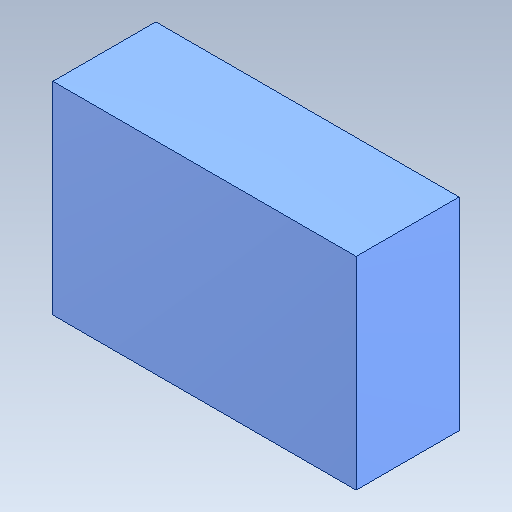
# Autodesk Inventor part: 100
Saved by Autodesk Inventor 2021 (Build 250183000, 183)
## iProperties
Created: 2020-11-03
Part Number: 100
Material: Generic
Document SubType Name: Modeling
Designer: faiya
Density: 1 g/cm^3
Appearance: R0603, 100
Author: faiya
Autodesk Inventor part; units mm, degrees
ref_plane "YZ Plane" through (0, 0, 0) normal (1, 0, 0) x (0, 1, 0)
ref_plane "XZ Plane" through (0, 0, 0) normal (0, 1, 0) x (-1, 0, 0)
ref_plane "XY Plane" through (0, 0, 0) normal (0, 0, 1) x (1, 0, 0)
sketch "R0603, 100_56" plane through (0, 0, 0) normal (0, 0, 1) x (1, 0, 0)
  line L0 (-1.473, 0.983) -> (1.473, 0.983)
  line L1 (1.473, 0.983) -> (1.473, -0.983)
  line L2 (1.473, -0.983) -> (-1.473, -0.983)
  line L3 (-1.473, -0.983) -> (-1.473, 0.983)
  constraints: 8 end point
extrude "Extrusion1" add sketch "R0603, 100_56" along normal blind 1
body "Solid1"
